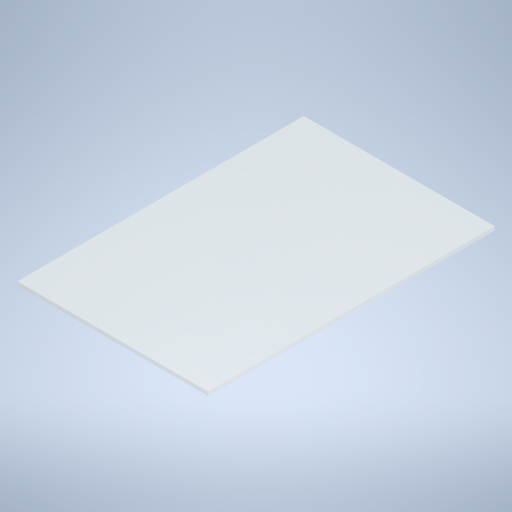
# Autodesk Inventor part: TurbineWindow
Saved by Autodesk Inventor 2024 (Build 280153000, 153)
## iProperties
Created: 2025-01-10
Part Number: TurbineWindow
Material: Glas
Document SubType Name: Modeling
Designer: maxho
Density: 2.18 g/cm^3
Appearance: Klar
Author: maxho
Autodesk Inventor part; units mm, degrees
ref_plane "YZ Plane" through (0, 0, 0) normal (1, 0, 0) x (0, 1, 0)
ref_plane "XZ Plane" through (0, 0, 0) normal (0, 1, 0) x (-1, 0, 0)
ref_plane "XY Plane" through (0, 0, 0) normal (0, 0, 1) x (1, 0, 0)
sketch "Skizze1" plane through (0, 0, 0) normal (0, 0, 1) x (1, 0, 0)
  line L0 (50, -75) -> (-50, -75)
  line L1 (-50, -75) -> (-50, 75)
  line L2 (-50, 75) -> (50, 75)
  line L3 (50, 75) -> (50, -75)
  line L4 (50, -75) -> (-50, 75) construction
  line L5 (-50, -75) -> (50, 75) construction
  point P0 (0, 0)
  dimension "d0" = 100
  dimension "d1" = 150
  constraints: 12 end point, 2 midpoint, 2 parallel, 1 horizontal, 1 perpendicular
  measures "d0" distance of L1.end L2.end
  measures "d1" distance of L0.end L1.end
extrude "Extrusion1" add sketch "Skizze1" along normal blind 2
